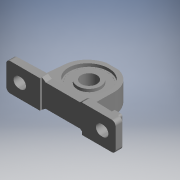
# Autodesk Inventor part: PDRM25_b
Saved by Autodesk Inventor 2017.3 (Build 213256000, 256)
## iProperties
Part Number: PDRM25_b
Material: Generic
Catalog Web Link: www.cadenas.de
Description: PDRM_body-Ball Bearing Units - Pillow Casting Housing Type -
Vendor: MISUMI
Document SubType Name: Modeling
Designer: partserver
Manufacturer: MISUMI
Mass: 209.573 g
Surface Area: 412.514 cm^2
Volume: 209.573 cm^3
Density: 1 g/cm^3
Appearance: PSOLRGB-175-175-175
Category: PARTsolutions
Company: MISUMI
Title: PDRM25
Author: Cadenas PARTsolutions
Comments: Ball Bearing Units - Pillow Casting Housing Type -
PSOL_IDENT_0: {$CADENAS_DATA\23d-libs\misumi\metric\12_bearing_holders\pdrm\pdrm_body.prj},157 {VTYP=3D},{NB=PDRM2
PSOL_IDENT_1: 5_b},{LINA=PDRM25},{NN=PDRM_body},{DATE=18.09.2019 02:28:40},{GEOMDATE=03.09.2019 08:48:32},{VERSION=
PSOL_IDENT_2: },{LINEID=10},{WBVAR=},{WBNUMERIC=}  {NB=PDRM25_b},{LINA=PDRM25},{KT=DUMMY},{PN=PDRM25},{TYPE=PDRM},
PSOL_IDENT_3: {MTH=Alloy Cast Iron Class No.30},{MTB=52100 Bearing Steel},{MTRS=Silicon Rubber},{MTSS=4137 Alloy S
PSOL_IDENT_4: teel},{PRECISION=JIS B 1558, JIS B 1559},{OT=-15 ~+100},{D=25},{JIS=UCP305},{H=45},{L=175},{L1=132},
PSOL_IDENT_5: {A=45},{DD1=20},{DD=17},{TT=16},{H1=84},{B=38},{S=15},{CRR=21.3},{COR=10.9},{M1=M6x0.75},{M1ALG=6},{
PSOL_IDENT_6: T=390},{ALC=1065},{MASS=1600},{HR1=39},{HR2=63},{HR3=58.335},{HR4=36.9},{HH1=11},{HH2=13},{HW2=55},{
PSOL_IDENT_7: HW3=67},{HW4=80.5},{HA1=2.186},{HW5=36.5},{HW6=29},{R1=3},{R2=15},{R3=6},{LEN1=82.5},{LEN2=15},{W=30
PSOL_IDENT_8: },{BW=21},{GZ=5.0},{LS=8}
NB: PDRM25_b
NN: PDRM_body
NT: Ball Bearing Units - Pillow Casting Housing Type -
NBSYN: $PN._b
LINA: PDRM25
CATALOG: Misumi
PN: PDRM25
TYPE: PDRM
MTH: Alloy Cast Iron Class No.30
MTB: 52100 Bearing Steel
MTRS: Silicon Rubber
MTSS: 4137 Alloy Steel
PRECISION: JIS B 1558, JIS B 1559
OT: -15 ~+100
D: 25
JIS: UCP305
H: 45
L: 175
L1: 132
A: 45
DD1: 20
DD: 17
TT: 16
H1: 84
B: 38
S: 15
CRR: 21.3
COR: 10.9
M1: M6x0.75
T: 390
ALC: 1065
MASS: 1600
SUPPLIER: MISUMI
ARTICLENO: PDRM25_b
BOMINFO: PDRM25
CREATOR: CADENAS GmbH
Autodesk Inventor part; units mm, degrees
sketch "_____1" plane through (0, 0, 0) normal (0, 0, 1) x (1, 0, 0)
  line L0 (-40.25, -32) -> (40.25, -32)
  line L1 (40.25, -32) -> (38.9717, 1.4875)
  arc A0 (38.9717, 1.4875) -> (-38.9717, 1.4875) centre (0, -0.0001) ccw
  line L2 (-38.9717, 1.4875) -> (-40.25, -32)
  constraints: 6 end point, 2 point on circle, 1 centre point
extrude "Extrusion1" add sketch "_____1" along normal mid plane 45
sketch "_____2" plane through (0, 0, 0) normal (1, 0, 0) x (0, 1, 0)
  line L0 (42, 22.5) -> (-32, 22.5)
  line L1 (-32, 22.5) -> (-32, 18.25)
  line L2 (-32, 18.25) -> (37.739, 14.5)
  arc A0 (37.739, -14.5) -> (37.739, 14.5) centre (-45, 0) ccw
  line L3 (37.739, -14.5) -> (-32, -18.25)
  line L4 (-32, -18.25) -> (-32, -22.5)
  line L5 (-32, -22.5) -> (42, -22.5)
  line L6 (42, -22.5) -> (42, 22.5)
  constraints: 14 end point, 2 point on circle, 1 centre point
extrude "Extrusion2" cut sketch "_____2" along normal mid plane 90
sketch "_____3" plane through (0, 0, 0) normal (0, 0, 1) x (1, 0, 0)
  line L0 (-87.5, -34) -> (-87.5, -45)
  line L1 (-87.5, -45) -> (87.5, -45)
  line L2 (87.5, -45) -> (87.5, -34)
  line L3 (87.5, -34) -> (27.5, -32)
  line L4 (27.5, -32) -> (-27.5, -32)
  line L5 (-27.5, -32) -> (-87.5, -34)
  constraints: 12 end point
extrude "Extrusion3" add sketch "_____3" along normal mid plane 45
sketch "_____4" plane through (0, -29, 0) normal (0, 1, 0) x (1, 0, 0)
  line L0 (0, -15) -> (64.5, -15)
  arc A0 (67.5, -18) -> (64.5, -15) centre (64.5, -18) ccw
  line L1 (67.5, -18) -> (67.5, -19.5)
  arc A1 (67.5, -19.5) -> (70.5, -22.5) centre (70.5, -19.5) ccw
  line L2 (70.5, -22.5) -> (79.5, -22.5)
  arc A2 (79.5, -22.5) -> (82.5, -19.5) centre (79.5, -19.5) ccw
  line L3 (82.5, -19.5) -> (82.5, 0)
  arc A3 (82.5, 0) -> (67.5, 15) centre (67.5, 0) ccw
  line L4 (67.5, 15) -> (0, 15)
  line L5 (0, 15) -> (0, -15)
  constraints: 12 end point, 8 point on circle, 4 centre point
extrude "Extrusion4" add sketch "_____4" against normal blind 16
sketch "_____5" plane through (0, -29, 0) normal (0, 1, 0) x (1, 0, 0)
  line L0 (-82.5, 19.5) -> (-82.5, 0)
  arc A0 (-82.5, 0) -> (-67.5, -15) centre (-67.5, 0) ccw
  line L1 (-67.5, -15) -> (0, -15)
  line L2 (0, -15) -> (0, 15)
  line L3 (0, 15) -> (-64.5, 15)
  arc A1 (-67.5, 18) -> (-64.5, 15) centre (-64.5, 18) ccw
  line L4 (-67.5, 18) -> (-67.5, 19.5)
  arc A2 (-67.5, 19.5) -> (-70.5, 22.5) centre (-70.5, 19.5) ccw
  line L5 (-70.5, 22.5) -> (-79.5, 22.5)
  arc A3 (-79.5, 22.5) -> (-82.5, 19.5) centre (-79.5, 19.5) ccw
  constraints: 12 end point, 8 point on circle, 4 centre point
extrude "Extrusion5" add sketch "_____5" against normal blind 16
sketch "_____6" plane through (0, -29, 0) normal (0, 1, 0) x (1, 0, 0)
  line L0 (-90.5, 25.5) -> (-90.5, -25.5)
  line L1 (-90.5, -25.5) -> (90.5, -25.5)
  line L2 (90.5, -25.5) -> (90.5, 25.5)
  line L3 (90.5, 25.5) -> (-90.5, 25.5)
  line L4 (-87.5, 16.5) -> (-87.5, -16.5)
  arc A0 (-87.5, -16.5) -> (-81.5, -22.5) centre (-81.5, -16.5) ccw
  line L5 (-81.5, -22.5) -> (-33.5, -22.5)
  line L6 (-33.5, -22.5) -> (-27.5, -18.25)
  line L7 (-27.5, -18.25) -> (27.5, -18.25)
  line L8 (27.5, -18.25) -> (33.5, -22.5)
  line L9 (33.5, -22.5) -> (81.5, -22.5)
  arc A1 (81.5, -22.5) -> (87.5, -16.5) centre (81.5, -16.5) ccw
  line L10 (87.5, -16.5) -> (87.5, 16.5)
  arc A2 (87.5, 16.5) -> (81.5, 22.5) centre (81.5, 16.5) ccw
  line L11 (81.5, 22.5) -> (33.5, 22.5)
  line L12 (33.5, 22.5) -> (27.5, 18.25)
  line L13 (27.5, 18.25) -> (-27.5, 18.25)
  line L14 (-27.5, 18.25) -> (-33.5, 22.5)
  line L15 (-33.5, 22.5) -> (-81.5, 22.5)
  arc A3 (-81.5, 22.5) -> (-87.5, 16.5) centre (-81.5, 16.5) ccw
  constraints: 32 end point, 8 point on circle, 4 centre point
extrude "Extrusion6" cut sketch "_____6" against normal blind 16
sketch "_____7" plane through (0, -29, 0) normal (0, 1, 0) x (1, 0, 0)
  arc A0 (64.5, 8.5) -> (64.5, -8.5) centre (64.5, 0) ccw
  line L0 (64.5, -8.5) -> (67.5, -8.5)
  arc A1 (67.5, -8.5) -> (67.5, 8.5) centre (67.5, 0) ccw
  line L1 (67.5, 8.5) -> (64.5, 8.5)
  constraints: 4 end point, 4 point on circle, 2 centre point
extrude "Extrusion7" cut sketch "_____7" against normal blind 16
sketch "_____8" plane through (0, -29, 0) normal (0, 1, 0) x (1, 0, 0)
  arc A0 (-67.5, 8.5) -> (-67.5, -8.5) centre (-67.5, 0) ccw
  line L0 (-67.5, -8.5) -> (-64.5, -8.5)
  arc A1 (-64.5, -8.5) -> (-64.5, 8.5) centre (-64.5, 0) ccw
  line L1 (-64.5, 8.5) -> (-67.5, 8.5)
  constraints: 4 end point, 4 point on circle, 2 centre point
extrude "Extrusion8" cut sketch "_____8" against normal blind 16
sketch "_____9" plane through (0, 0, 0) normal (1, 0, 0) x (0, 1, 0)
  line L0 (0, -21) -> (0, -10.5)
  line L1 (0, -10.5) -> (31.5, -10.5)
  line L2 (31.5, -10.5) -> (31.5, -21)
  line L3 (31.5, -21) -> (0, -21)
  line L4 (0, -21) -> (0, -10.5)
  constraints: 10 end point
revolve "Revolution1" cut sketch "_____9" angle 360 about axis through (0, 0, -21) along (0, 0, -1)
sketch "_____10" plane through (0, 0, 0) normal (1, 0, 0) x (0, 1, 0)
  line L0 (0, 10.5) -> (0, 21)
  line L1 (0, 21) -> (31.5, 21)
  line L2 (31.5, 21) -> (31.5, 10.5)
  line L3 (31.5, 10.5) -> (0, 10.5)
  line L4 (0, 10.5) -> (0, 21)
  constraints: 10 end point
revolve "Revolution2" cut sketch "_____10" angle 360 about axis through (0, 0, 10.5) along (0, 0, -1)
sketch "_____11" plane through (0, 0, 0) normal (1, 0, 0) x (0, 1, 0)
  line L0 (0, -50) -> (0, 50)
  arc A0 (29.2175, -10.5) -> (29.1175, -10.5) centre (29.1675, -10.5) ccw
  line L1 (29.1175, -10.5) -> (29.2175, -10.5)
  constraints: 4 end point, 2 point on circle, 1 centre point
revolve "Revolution3" cut sketch "_____11" angle 360 about axis through (0, 0, -50) along (0, 0, -1)
sketch "_____12" plane through (0, 0, 0) normal (1, 0, 0) x (0, 1, 0)
  line L0 (0, -50) -> (0, 50)
  line L1 (29.2175, 10.5) -> (29.1175, 10.5)
  arc A0 (29.1175, 10.5) -> (29.2175, 10.5) centre (29.1675, 10.5) ccw
  constraints: 4 end point, 2 point on circle, 1 centre point
revolve "Revolution4" cut sketch "_____12" angle 360 about axis through (0, 0, -50) along (0, 0, -1)
sketch "_____13" plane through (0, 0, 0) normal (1, 0, 0) x (0, 1, 0)
  line L0 (0, -15) -> (0, 23)
  line L1 (0, 23) -> (18.45, 23)
  line L2 (18.45, 23) -> (18.45, -15)
  line L3 (18.45, -15) -> (0, -15)
  line L4 (0, -15) -> (0, 23)
  constraints: 10 end point
revolve "Revolution5" add sketch "_____13" angle 360 about axis through (0, 0, -15) along (0, 0, -1)
sketch "Sketch14" plane through (0, 0, -15) normal (0, 0, -1) x (-1, 0, 0)
  point P0 (0, 0)
hole "Hole1" at (0, 0, -15) direction (0, 0, 1) diameter 25 depth 38
sketch "_____15" plane through (0, 0, 0) normal (1, 0, 0) x (0, 1, 0)
  line L0 (12, 17) -> (18.45, 17)
  line L1 (18.45, 17) -> (18.45, 14)
  line L2 (18.45, 14) -> (17.9085, 14.5415)
  line L3 (17.9085, 14.5415) -> (12, 14.5415)
  line L4 (12, 14.5415) -> (12, 17)
  line L5 (12, 17) -> (18.45, 17)
  constraints: 12 end point
revolve "Revolution6" cut sketch "_____15" angle 360 about axis through (0, 12, 17) along (0, -1, 0)
thread "Thread1" size "M6x1" class "6H" standard "ISO Metric profile" length 5.4085
sketch "_____16" plane through (0, 0, 0) normal (-0.5, 0.8660254, 0) x (0, 0, -1)
  line L0 (-17, 12) -> (-17, 18.45)
  line L1 (-17, 18.45) -> (-14, 18.45)
  line L2 (-14, 18.45) -> (-14.5415, 17.9085)
  line L3 (-14.5415, 17.9085) -> (-14.5415, 12)
  line L4 (-14.5415, 12) -> (-17, 12)
  line L5 (-17, 12) -> (-17, 18.45)
  constraints: 12 end point
revolve "Revolution7" cut sketch "_____16" angle 360 about axis through (-10.3923, -6, 17) along (0.8660254, 0.5, 0)
thread "Thread2" size "M6x1" class "6H" standard "ISO Metric profile" length 5.4085
sketch "_____19" plane through (0, 0, 5) normal (0, 0, 1) x (1, 0, 0)
  line L0 (0, 48.1) -> (0, 38.25)
  line L1 (0, 38.25) -> (-3.3, 38.25)
  line L2 (-3.3, 38.25) -> (-3.3, 39.5)
  line L3 (-3.3, 39.5) -> (-3.5, 39.5)
  line L4 (-3.5, 39.5) -> (-5.2321, 40.5)
  line L5 (-5.2321, 40.5) -> (-3.5, 41.5)
  arc A0 (-3.5, 41.5) -> (-2.853, 43.2508) centre (-8.736, 44.4299) ccw
  arc A1 (-2.853, 43.2508) -> (-2.9276, 43.7772) centre (-3.6374, 43.4081) ccw
  arc A2 (-3.3, 45.3) -> (-2.9276, 43.7772) centre (0, 45.3) ccw
  line L6 (-3.3, 45.3) -> (-2.4, 48)
  line L7 (-2.4, 48) -> (-0.5546, 48)
  arc A3 (0, 48.1) -> (-0.5546, 48) centre (0, 46.512) ccw
  line L8 (0, 48.1) -> (0, 38.25)
  constraints: 18 end point, 8 point on circle, 4 centre point
revolve "Revolution8" add sketch "_____19" angle 360 about axis through (0, 48.1, 5) along (0, 1, 0)
sketch "_____20" plane through (0, 39, 0) normal (0, 1, 0) x (1, 0, 0)
  circle A0 centre (0, -5) radius 10
  line L0 (-4.0415, -5) -> (-2.0207, -8.5)
  line L1 (-2.0207, -8.5) -> (2.0207, -8.5)
  line L2 (2.0207, -8.5) -> (4.0415, -5)
  line L3 (4.0415, -5) -> (2.0207, -1.5)
  line L4 (2.0207, -1.5) -> (-2.0207, -1.5)
  line L5 (-2.0207, -1.5) -> (-4.0415, -5)
  constraints: 12 end point, 1 centre point
extrude "Extrusion9" cut sketch "_____20" along normal blind 4
sketch "_____21" plane through (0, 0, 0) normal (0, 0, 1) x (1, 0, 0)
  line L0 (-33.5, -42) -> (-33.5, -45)
  line L1 (-33.5, -45) -> (33.5, -45)
  line L2 (33.5, -45) -> (33.5, -42)
  line L3 (33.5, -42) -> (-33.5, -42)
  constraints: 8 end point
extrude "Extrusion10" cut sketch "_____21" along normal mid plane 90
ref_plane "cp1_XY" through (0, 12.5, 17) normal (0, 1, 0) x (1, 0, 0)
ref_plane "cp1_YZ" through (0, 12.5, 17) normal (1, 0, 0) x (0, 0, -1)
ref_plane "cp1_ZX" through (0, 12.5, 17) normal (0, 0, -1) x (0, 1, 0)
ref_plane "cp2_XY" through (-10.8253, -6.25, 17) normal (-0.8660254, -0.5, 0) x (-0.5, 0.8660254, 0)
ref_plane "cp2_YZ" through (-10.8253, -6.25, 17) normal (-0.5, 0.8660254, 0) x (0, 0, -1)
ref_plane "cp2_ZX" through (-10.8253, -6.25, 17) normal (0, 0, -1) x (-0.8660254, -0.5, 0)
body "Solid1"
